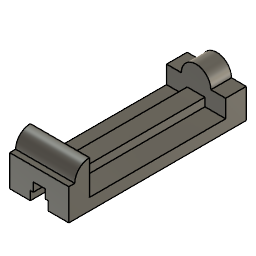
Task3B (Autodesk Fusion 360 design; units mm, degrees)
part number: 2026-03-02-09-39-55-885
Autodesk Fusion 360 part; units mm, degrees
note: some values were not read from the file. Set by a fixed rule: which face or edge a step refers to.
sketch "Sketch1" plane through (0, 0, 0) normal (0, 1, 0) x (1, 0, 0)
  line L0 (-50, 0) -> (50, 0)
  line L1 (50, 0) -> (50, -50)
  line L2 (50, -50) -> (-50, -50)
  line L3 (-50, -50) -> (-50, 0)
  constraint horizontal L0
  constraint vertical L1
  constraint horizontal L2
  constraint vertical L3
extrude "Extrude1" add sketch "Sketch1" along normal blind 300
sketch "Sketch2" plane through (0, 0, 0) normal (0, -1, 0) x (1, 0, 0)
  line L0 (50, 50) -> (-50, 50)
  line L1 (-50, 50) -> (-50, 0)
  line L2 (-50, 0) -> (50, 0)
  line L3 (50, 0) -> (50, 50)
  line L4 (-15, 0) -> (-15, 15)
  line L5 (-15, 15) -> (-10, 15)
  line L6 (-10, 15) -> (-10, 30)
  line L7 (-10, 30) -> (10, 30)
  line L8 (10, 30) -> (10, 15)
  line L9 (10, 15) -> (15, 15)
  line L10 (15, 15) -> (15, 0)
  constraint coincident L2 L4.start
  constraint perpendicular L2 L4
  constraint perpendicular L4 L5
  constraint perpendicular L5 L6
  constraint perpendicular L6 L7
  constraint perpendicular L7 L8
  constraint perpendicular L8 L9
  constraint coincident L2 L10.end
  constraint perpendicular L2 L10
extrude "Extrude2" cut sketch "Sketch2" against normal blind 460 contours L2 L4 L5 L6 L7 L8 L9 L10
sketch "Sketch3" plane through (0, 0, 50) normal (0, 0, 1) x (-1, 0, 0)
  line L0 (50, 0) -> (-50, 0)
  line L1 (-50, 0) -> (-50, -300)
  line L2 (-50, -300) -> (50, -300)
  line L3 (50, -300) -> (50, 0)
  line L4 (50, 0) -> (15, 0)
  line L5 (15, -300) -> (50, -300)
  line L6 (15, 0) -> (15, -300)
  constraint coincident L0.start L3.end
  constraint coincident L0 L4.end
  constraint coincident L2 L5.start
  constraint coincident L2.end L3.start
  constraint perpendicular L5 L6
extrude "Extrude3" cut sketch "Sketch3" against normal blind 30 contours L0 L2 L3 L4 L5 L6
sketch "Sketch4" plane through (0, 0, 50) normal (0, 0, 1) x (-1, 0, 0)
  line L0 (15, -300) -> (15, 0)
  line L1 (15, 0) -> (-50, 0)
  line L2 (-50, 0) -> (-50, -300)
  line L3 (-50, -300) -> (15, -300)
  line L4 (-15, 0) -> (-15, -300)
  constraint coincident L1 L4.start
  constraint coincident L3 L4.end
  constraint perpendicular L3 L4
extrude "Extrude4" cut sketch "Sketch4" against normal blind 30 contours L1 L2 L3 L4
extrude "Extrude5" cut 1 faces at (5, 100, 50) along direction (0, 0, -1) blind 16
sketch "Sketch5" plane through (0, 0, 34) normal (0, 0, 1) x (-1, 0, 0)
  line L0 (-15, 0) -> (-15, -300)
  line L1 (-15, -300) -> (15, -300)
  line L2 (15, -300) -> (15, 0)
  line L3 (15, 0) -> (-15, 0)
  line L4 (50, -5) -> (15, -5)
  line L5 (15, -5) -> (-15, -5)
  line L6 (-15, -5) -> (-50, -5)
  constraint coincident L2 L4.end
  constraint perpendicular L2 L4
  constraint coincident L0 L5.end
  constraint perpendicular L0 L5
  constraint perpendicular L0 L6
extrude "Extrude6" add sketch "Sketch5" along normal blind 24 contours L0 L2 L3 L5
sketch "Sketch6" plane through (-15, 0, 0) normal (-1, 0, 0) x (0, -1, 0)
  line L0 (-5, 34) -> (-300, 34)
  line L1 (-300, 34) -> (-300, 20)
  line L2 (-300, 20) -> (0, 20)
  line L3 (0, 20) -> (0, 58)
  line L4 (0, 58) -> (-5, 58)
  line L5 (-5, 58) -> (-5, 34)
  line L6 (-5, 34) -> (-5, 20)
  constraint coincident L0.start L5.end
  constraint coincident L2 L6.end
  constraint perpendicular L2 L6
extrude "Extrude7" add sketch "Sketch6" along normal blind 35 contours L2 L3 L4 L5 L6
sketch "Sketch7" plane through (15, 0, 0) normal (1, 0, 0) x (0, 1, 0)
  line L0 (300, 34) -> (5, 34)
  line L1 (5, 34) -> (5, 58)
  line L2 (5, 58) -> (0, 58)
  line L3 (0, 58) -> (0, 20)
  line L4 (0, 20) -> (300, 20)
  line L5 (300, 20) -> (300, 34)
  line L6 (5, 34) -> (5, 20)
  constraint coincident L0.end L1.start
  constraint coincident L4 L6.end
  constraint perpendicular L4 L6
extrude "Extrude8" add sketch "Sketch7" along normal blind 35 contours L1 L2 L3 L4 L6
extrude "Extrude9" cut 1 faces at (16.6667, 1.6667, 58) along direction (0, 0, -1) blind 5
extrude "Extrude10" add 1 faces at (38.3333, 5, 35.6667) along direction (0, 1, 0) blind 30
sketch "Sketch8" plane through (0, 0, 53) normal (0, 0, 1) x (-1, 0, 0)
  line L0 (50, 0) -> (-50, 0)
  line L1 (-50, 0) -> (-50, -35)
  line L2 (-50, -35) -> (50, -35)
  line L3 (50, -35) -> (50, 0)
  line L4 (-50, -10) -> (50, -10)
  constraint coincident L1 L4.start
  constraint coincident L3 L4.end
  constraint perpendicular L3 L4
extrude "Extrude11" add sketch "Sketch8" along normal blind 25 contours L1 L2 L3 L4
sketch "Sketch9" plane through (50, 0, 0) normal (1, 0, 0) x (0, 1, 0)
  line L0 (10, 53) -> (0, 53)
  line L1 (0, 53) -> (0, 0)
  line L2 (0, 0) -> (300, 0)
  line L3 (300, 0) -> (300, 20)
  line L4 (300, 20) -> (35, 20)
  line L5 (35, 20) -> (35, 78)
  line L6 (35, 78) -> (10, 78)
  line L7 (10, 78) -> (10, 53)
  circle A0 centre (35, 53) radius 25
  constraint coincident L5 A0.centre
  constraint coincident L0.start A0
extrude "Extrude12" cut sketch "Sketch9" against normal blind 175 contours L6 L7 A0
extrude "Extrude13" cut 1 faces at (-38.3333, 300, 11.6667) along direction (0, -1, 0) blind 150
mirror "Mirror1" about plane through (0, 150, 0) normal (0, 1, 0) of bodies 1 merged
extrude "Extrude14" add 1 faces at (-16.6667, 296.6667, 53) along direction (0, 0, 1) blind 30
extrude "Extrude15" cut 1 faces at (16.6667, 290, 63) along direction (0, -1, 0) blind 30
extrude "Extrude16" add 1 faces at (16.6667, 290, 63) along direction (0, -1, 0) blind 25
sketch "Sketch10" plane through (0, 300, 0) normal (0, 1, 0) x (-1, 0, 0)
  line L0 (-50, 83) -> (-50, 0)
  line L1 (-50, 0) -> (-15, 0)
  line L2 (-15, 0) -> (-15, 15)
  line L3 (-15, 15) -> (-10, 15)
  line L4 (-10, 15) -> (-10, 30)
  line L5 (-10, 30) -> (10, 30)
  line L6 (10, 30) -> (10, 15)
  line L7 (10, 15) -> (15, 15)
  line L8 (15, 15) -> (15, 0)
  line L9 (15, 0) -> (50, 0)
  line L10 (50, 0) -> (50, 83)
  line L11 (50, 83) -> (-50, 83)
  line L12 (0, 30) -> (0, 50)
  line L13 (0, 50) -> (-50, 50)
  line L14 (0, 50) -> (50, 50)
  circle A0 centre (0, 50) radius 25
  constraint midpoint L5 L12.start
  constraint perpendicular L5 L12
  constraint coincident L0 L13.end
  constraint perpendicular L0 L13
  constraint coincident L10 L14.end
  constraint perpendicular L10 L14
  constraint coincident L12.end L13.start
extrude "Extrude17" cut sketch "Sketch10" against normal blind 45 contours L0 L10 L11 L13 L14 A0
